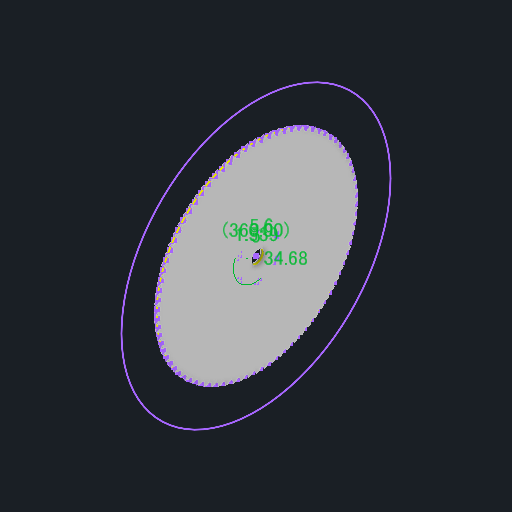
# Autodesk Inventor part: 25A80_()
Saved by Autodesk Inventor 2025.2 (Build 292293000, 293)
## iProperties
Category: PARTsolutions
Company: KANA
Created: 2025-03-15
Part Number: 25A80_()
Material: Generic
Catalog Web Link: www.cadenas.de
Description: 25A-Un-finished
Vendor: KANA
Document SubType Name: Modeling
Designer: psAdmin
Manufacturer: KANA
Mass: 58.7278 g
Surface Area: 427.105 cm^2
Volume: 58.7278 cm^3
Density: 1 g/cm^3
Appearance: PSOLRGB-175-175-175
PSOL_IDENT_0: {$CADENAS_DATA/23d-libs/kana/sprockets/chain_no_25/un_finished_sprocket_steel/a_type/25a.prj},156 {V
PSOL_IDENT_1: TYP=3D},{NB=25A80_()},{LINA=25A80},{NN=25A},{DATE=07.03.2025 00:51:20},{GEOMDATE=20.11.2024 07:31:23
PSOL_IDENT_2: },{VERSION=},{LINEID=550},{WBVAR=SURFT},{WBNUMERIC=}  {NB=25A80_()},{LINA=25A80},{KT=DUMMY},{ORDERNO=
PSOL_IDENT_3: 25A80},{TYPE=25A},{NOT=80},{NOTX=80.000},{DP=161.74},{DC=158.44},{DC2=158.44},{DO=165},{T=2.9},{DR=3
PSOL_IDENT_4: .300},{MAT=None},{MATC=},{SD=11},{SURFT=},{SURFTNB=},{DCX2=0},{CAUTION=The tooth profile in the CAD
PSOL_IDENT_5: models differ from the actual shape.}
NB: 25A80_()
NN: 25A
NT: Un-finished
NBSYN: 25A$NOT._($SURFT.)
LINA: 25A80
CATALOG: KANA
TYPE: 25A
NOT: 80
DP: 161.74
DC: 158.44
DC2: 158.44
DO: 165
T: 2.9
SD: 11
SURFT: No symbol : No
CAUTION: The tooth profile in the CAD models differ from the actual shape.
SUPPLIER: KANA
ARTICLENO: 25A80_()
BOMINFO: 25A80
CREATOR: CADENAS GmbH
Title: 25A80
Author: Cadenas PARTsolutions
Comments: Un-finished
Autodesk Inventor part; units mm, degrees
sketch "Sketch_1" plane through (0, 0, 0) normal (0, 0, 1) x (1, 0, 0)
  line L0 (2.9, 0) -> (0, 0)
  line L1 (0, 5.5) -> (2.9, 5.5)
  line L2 (2.9, 5.5) -> (2.9, 81.2642)
  arc A0 (2.9, 81.2642) -> (2.175, 82.5) centre (-0.241, 80.2521) ccw
  line L3 (2.175, 82.5) -> (0.725, 82.5)
  arc A1 (0.725, 82.5) -> (0, 81.2642) centre (3.141, 80.2521) ccw
  line L4 (0, 81.2642) -> (0, 5.5)
  constraints: 10 end point, 4 point on circle, 2 centre point
revolve "Revolution1" add sketch "Sketch_1" angle 360 about axis through (2.9, 0, 0) along (1, 0, 0)
sketch "Sketch_2" plane through (1.45, 0, 0) normal (1, 0, 0) x (0, 0, -1)
  circle A0 centre (0, -0.0001) radius 110
  arc A1 (-82.4999, 0.15) -> (-82.4999, -0.15) centre (0, -0.0001) ccw
  line L0 (-82.4999, -0.15) -> (-79.9248, -1.781)
  arc A2 (-79.8181, -4.4953) -> (-79.9248, -1.781) centre (-80.8077, -3.1749) ccw
  line L1 (-79.8181, -4.4953) -> (-82.2573, -6.3233)
  arc A3 (-82.2573, -6.3233) -> (-82.2338, -6.6224) centre (0, 0) ccw
  line L2 (-82.2338, -6.6224) -> (-79.5386, -8.0464)
  arc A4 (-79.2194, -10.7439) -> (-79.5386, -8.0464) centre (-80.3094, -9.5052) ccw
  line L3 (-79.2194, -10.7439) -> (-81.5076, -12.7577)
  arc A5 (-81.5076, -12.7577) -> (-81.4607, -13.054) centre (0, 0) ccw
  line L4 (-81.4607, -13.054) -> (-78.6621, -14.2621)
  arc A6 (-78.1322, -16.9263) -> (-78.6621, -14.2621) centre (-79.3161, -15.777) ccw
  line L5 (-78.1322, -16.9263) -> (-80.2554, -19.1134)
  arc A7 (-80.2554, -19.1134) -> (-80.1854, -19.4051) centre (0, 0) ccw
  line L6 (-80.1854, -19.4051) -> (-77.3007, -20.3899)
  arc A8 (-76.5633, -23.0043) -> (-77.3007, -20.3899) centre (-77.8338, -21.9514) ccw
  line L7 (-76.5633, -23.0043) -> (-78.5084, -25.3512)
  arc A9 (-78.5084, -25.3512) -> (-78.4157, -25.6365) centre (0, 0) ccw
  line L8 (-78.4157, -25.6365) -> (-75.4626, -26.392)
  arc A10 (-74.5224, -28.9404) -> (-75.4626, -26.392) centre (-75.8715, -27.9905) ccw
  line L9 (-74.5224, -28.9404) -> (-76.2773, -31.4327)
  arc A11 (-76.2773, -31.4327) -> (-76.1625, -31.7099) centre (0, 0) ccw
  line L10 (-76.1625, -31.7099) -> (-73.1593, -32.2313)
  arc A12 (-72.0221, -34.6982) -> (-73.1593, -32.2313) centre (-73.4415, -33.857) ccw
  line L11 (-72.0221, -34.6982) -> (-73.576, -37.3205)
  arc A13 (-73.576, -37.3205) -> (-73.4398, -37.5878) centre (0, 0) ccw
  line L12 (-73.4398, -37.5878) -> (-70.4049, -37.872)
  arc A14 (-69.0776, -40.242) -> (-70.4049, -37.872) centre (-70.5588, -39.5148) ccw
  line L13 (-69.0776, -40.242) -> (-70.4211, -42.9782)
  arc A15 (-70.4211, -42.9782) -> (-70.2643, -43.234) centre (0, 0) ccw
  line L14 (-70.2643, -43.234) -> (-67.2165, -43.2791)
  arc A16 (-65.7074, -45.5377) -> (-67.2165, -43.2791) centre (-67.2409, -44.929) ccw
  line L15 (-65.7074, -45.5377) -> (-66.832, -48.3709)
  arc A17 (-66.832, -48.3709) -> (-66.6556, -48.6136) centre (0, 0) ccw
  line L16 (-66.6556, -48.6136) -> (-63.6136, -48.4195)
  arc A18 (-61.932, -50.5527) -> (-63.6136, -48.4195) centre (-63.5086, -50.0661) ccw
  line L17 (-61.932, -50.5527) -> (-62.8308, -53.4653)
  arc A19 (-62.8308, -53.4653) -> (-62.636, -53.6934) centre (0, 0) ccw
  line L18 (-62.636, -53.6934) -> (-59.6186, -53.2613)
  arc A20 (-57.7747, -55.256) -> (-59.6186, -53.2613) centre (-59.3847, -54.8946) ccw
  line L19 (-57.7747, -55.256) -> (-58.4423, -58.2301)
  arc A21 (-58.4423, -58.2301) -> (-58.2301, -58.4423) centre (0, 0) ccw
  line L20 (-58.2301, -58.4423) -> (-55.256, -57.7747)
  arc A22 (-53.2613, -59.6186) -> (-55.256, -57.7747) centre (-54.8946, -59.3847) ccw
  line L21 (-53.2613, -59.6186) -> (-53.6934, -62.636)
  arc A23 (-53.6934, -62.636) -> (-53.4653, -62.8308) centre (0, 0) ccw
  line L22 (-53.4653, -62.8308) -> (-50.5527, -61.932)
  arc A24 (-48.4195, -63.6136) -> (-50.5527, -61.932) centre (-50.0661, -63.5086) ccw
  line L23 (-48.4195, -63.6136) -> (-48.6136, -66.6556)
  arc A25 (-48.6136, -66.6556) -> (-48.3709, -66.832) centre (0, 0) ccw
  line L24 (-48.3709, -66.832) -> (-45.5377, -65.7074)
  arc A26 (-43.2791, -67.2165) -> (-45.5377, -65.7074) centre (-44.929, -67.2409) ccw
  line L25 (-43.2791, -67.2165) -> (-43.234, -70.2643)
  arc A27 (-43.234, -70.2643) -> (-42.9782, -70.4211) centre (0, 0) ccw
  line L26 (-42.9782, -70.4211) -> (-40.242, -69.0776)
  arc A28 (-37.872, -70.4049) -> (-40.242, -69.0776) centre (-39.5148, -70.5588) ccw
  line L27 (-37.872, -70.4049) -> (-37.5878, -73.4398)
  arc A29 (-37.5878, -73.4398) -> (-37.3205, -73.576) centre (0, 0) ccw
  line L28 (-37.3205, -73.576) -> (-34.6982, -72.0221)
  arc A30 (-32.2313, -73.1593) -> (-34.6982, -72.0221) centre (-33.857, -73.4415) ccw
  line L29 (-32.2313, -73.1593) -> (-31.7099, -76.1625)
  arc A31 (-31.7099, -76.1625) -> (-31.4327, -76.2773) centre (0, 0) ccw
  line L30 (-31.4327, -76.2773) -> (-28.9404, -74.5224)
  arc A32 (-26.392, -75.4626) -> (-28.9404, -74.5224) centre (-27.9905, -75.8715) ccw
  line L31 (-26.392, -75.4626) -> (-25.6365, -78.4157)
  arc A33 (-25.6365, -78.4157) -> (-25.3512, -78.5084) centre (0, 0) ccw
  line L32 (-25.3512, -78.5084) -> (-23.0043, -76.5633)
  arc A34 (-20.3899, -77.3007) -> (-23.0043, -76.5633) centre (-21.9514, -77.8338) ccw
  line L33 (-20.3899, -77.3007) -> (-19.4051, -80.1854)
  arc A35 (-19.4051, -80.1854) -> (-19.1134, -80.2554) centre (0, 0) ccw
  line L34 (-19.1134, -80.2554) -> (-16.9263, -78.1322)
  arc A36 (-14.2621, -78.6621) -> (-16.9263, -78.1322) centre (-15.777, -79.3161) ccw
  line L35 (-14.2621, -78.6621) -> (-13.054, -81.4607)
  arc A37 (-13.054, -81.4607) -> (-12.7577, -81.5076) centre (0, 0) ccw
  line L36 (-12.7577, -81.5076) -> (-10.7439, -79.2194)
  arc A38 (-8.0464, -79.5386) -> (-10.7439, -79.2194) centre (-9.5052, -80.3094) ccw
  line L37 (-8.0464, -79.5386) -> (-6.6224, -82.2338)
  arc A39 (-6.6224, -82.2338) -> (-6.3233, -82.2573) centre (0, 0) ccw
  line L38 (-6.3233, -82.2573) -> (-4.4953, -79.8181)
  arc A40 (-1.781, -79.9248) -> (-4.4953, -79.8181) centre (-3.1749, -80.8077) ccw
  line L39 (-1.781, -79.9248) -> (-0.15, -82.4999)
  arc A41 (-0.15, -82.4999) -> (0.15, -82.4999) centre (0, 0) ccw
  line L40 (0.15, -82.4999) -> (1.781, -79.9248)
  arc A42 (4.4953, -79.8181) -> (1.781, -79.9248) centre (3.1749, -80.8077) ccw
  line L41 (4.4953, -79.8181) -> (6.3233, -82.2573)
  arc A43 (6.3233, -82.2573) -> (6.6224, -82.2338) centre (0, 0) ccw
  line L42 (6.6224, -82.2338) -> (8.0464, -79.5386)
  arc A44 (10.7439, -79.2194) -> (8.0464, -79.5386) centre (9.5052, -80.3094) ccw
  line L43 (10.7439, -79.2194) -> (12.7577, -81.5076)
  arc A45 (12.7577, -81.5076) -> (13.054, -81.4607) centre (0, 0) ccw
  line L44 (13.054, -81.4607) -> (14.2621, -78.6621)
  arc A46 (16.9263, -78.1322) -> (14.2621, -78.6621) centre (15.777, -79.3161) ccw
  line L45 (16.9263, -78.1322) -> (19.1134, -80.2554)
  arc A47 (19.1134, -80.2554) -> (19.4051, -80.1854) centre (0, 0) ccw
  line L46 (19.4051, -80.1854) -> (20.3899, -77.3007)
  arc A48 (23.0043, -76.5633) -> (20.3899, -77.3007) centre (21.9514, -77.8338) ccw
  line L47 (23.0043, -76.5633) -> (25.3512, -78.5084)
  arc A49 (25.3512, -78.5084) -> (25.6365, -78.4157) centre (0, 0) ccw
  line L48 (25.6365, -78.4157) -> (26.392, -75.4626)
  arc A50 (28.9404, -74.5224) -> (26.392, -75.4626) centre (27.9905, -75.8715) ccw
  line L49 (28.9404, -74.5224) -> (31.4327, -76.2773)
  arc A51 (31.4327, -76.2773) -> (31.7099, -76.1625) centre (0, 0) ccw
  line L50 (31.7099, -76.1625) -> (32.2313, -73.1593)
  arc A52 (34.6982, -72.0221) -> (32.2313, -73.1593) centre (33.857, -73.4415) ccw
  line L51 (34.6982, -72.0221) -> (37.3205, -73.576)
  arc A53 (37.3205, -73.576) -> (37.5878, -73.4398) centre (0, 0) ccw
  line L52 (37.5878, -73.4398) -> (37.872, -70.4049)
  arc A54 (40.242, -69.0776) -> (37.872, -70.4049) centre (39.5148, -70.5588) ccw
  line L53 (40.242, -69.0776) -> (42.9782, -70.4211)
  arc A55 (42.9782, -70.4211) -> (43.234, -70.2643) centre (0, 0) ccw
  line L54 (43.234, -70.2643) -> (43.2791, -67.2165)
  arc A56 (45.5377, -65.7074) -> (43.2791, -67.2165) centre (44.929, -67.2409) ccw
  line L55 (45.5377, -65.7074) -> (48.3709, -66.832)
  arc A57 (48.3709, -66.832) -> (48.6136, -66.6556) centre (0, 0) ccw
  line L56 (48.6136, -66.6556) -> (48.4195, -63.6136)
  arc A58 (50.5527, -61.932) -> (48.4195, -63.6136) centre (50.0661, -63.5086) ccw
  line L57 (50.5527, -61.932) -> (53.4653, -62.8308)
  arc A59 (53.4653, -62.8308) -> (53.6934, -62.636) centre (0, 0) ccw
  line L58 (53.6934, -62.636) -> (53.2613, -59.6186)
  arc A60 (55.256, -57.7747) -> (53.2613, -59.6186) centre (54.8946, -59.3847) ccw
  line L59 (55.256, -57.7747) -> (58.2301, -58.4423)
  arc A61 (58.2301, -58.4423) -> (58.4423, -58.2301) centre (0, 0) ccw
  line L60 (58.4423, -58.2301) -> (57.7747, -55.256)
  arc A62 (59.6186, -53.2613) -> (57.7747, -55.256) centre (59.3847, -54.8946) ccw
  line L61 (59.6186, -53.2613) -> (62.636, -53.6934)
  arc A63 (62.636, -53.6934) -> (62.8308, -53.4653) centre (0, 0) ccw
  line L62 (62.8308, -53.4653) -> (61.9319, -50.5527)
  arc A64 (63.6136, -48.4195) -> (61.9319, -50.5527) centre (63.5086, -50.0661) ccw
  line L63 (63.6136, -48.4195) -> (66.6556, -48.6136)
  arc A65 (66.6556, -48.6136) -> (66.832, -48.3709) centre (0, 0) ccw
  line L64 (66.832, -48.3709) -> (65.7074, -45.5377)
  arc A66 (67.2165, -43.2791) -> (65.7074, -45.5377) centre (67.2409, -44.929) ccw
  line L65 (67.2165, -43.2791) -> (70.2643, -43.234)
  arc A67 (70.2643, -43.234) -> (70.4211, -42.9782) centre (0, 0) ccw
  line L66 (70.4211, -42.9782) -> (69.0776, -40.242)
  arc A68 (70.4049, -37.872) -> (69.0776, -40.242) centre (70.5588, -39.5148) ccw
  line L67 (70.4049, -37.872) -> (73.4398, -37.5878)
  arc A69 (73.4398, -37.5878) -> (73.576, -37.3205) centre (0, 0) ccw
  line L68 (73.576, -37.3205) -> (72.0221, -34.6982)
  arc A70 (73.1593, -32.2313) -> (72.0221, -34.6982) centre (73.4415, -33.857) ccw
  line L69 (73.1593, -32.2313) -> (76.1625, -31.7099)
  arc A71 (76.1625, -31.7099) -> (76.2773, -31.4327) centre (0, 0) ccw
  line L70 (76.2773, -31.4327) -> (74.5224, -28.9404)
  arc A72 (75.4626, -26.392) -> (74.5224, -28.9404) centre (75.8715, -27.9905) ccw
  line L71 (75.4626, -26.392) -> (78.4157, -25.6365)
  arc A73 (78.4157, -25.6365) -> (78.5084, -25.3512) centre (0, 0) ccw
  line L72 (78.5084, -25.3512) -> (76.5633, -23.0043)
  arc A74 (77.3007, -20.3899) -> (76.5633, -23.0043) centre (77.8338, -21.9514) ccw
  line L73 (77.3007, -20.3899) -> (80.1854, -19.4051)
  arc A75 (80.1854, -19.4051) -> (80.2554, -19.1134) centre (0, 0) ccw
  line L74 (80.2554, -19.1134) -> (78.1322, -16.9263)
  arc A76 (78.6621, -14.2621) -> (78.1322, -16.9263) centre (79.3161, -15.777) ccw
  line L75 (78.6621, -14.2621) -> (81.4607, -13.054)
  arc A77 (81.4607, -13.054) -> (81.5076, -12.7577) centre (0, 0) ccw
  line L76 (81.5076, -12.7577) -> (79.2194, -10.7439)
  arc A78 (79.5386, -8.0464) -> (79.2194, -10.7439) centre (80.3094, -9.5052) ccw
  line L77 (79.5386, -8.0464) -> (82.2338, -6.6224)
  arc A79 (82.2338, -6.6224) -> (82.2573, -6.3233) centre (0, 0) ccw
  line L78 (82.2573, -6.3233) -> (79.8181, -4.4953)
  arc A80 (79.9248, -1.781) -> (79.8181, -4.4953) centre (80.8077, -3.1749) ccw
  line L79 (79.9248, -1.781) -> (82.4999, -0.15)
  arc A81 (82.4999, -0.15) -> (82.4999, 0.15) centre (0, 0) ccw
  line L80 (82.4999, 0.15) -> (79.9248, 1.781)
  arc A82 (79.8181, 4.4953) -> (79.9248, 1.781) centre (80.8077, 3.1749) ccw
  line L81 (79.8181, 4.4953) -> (82.2573, 6.3233)
  arc A83 (82.2573, 6.3233) -> (82.2338, 6.6224) centre (0, 0) ccw
  line L82 (82.2338, 6.6224) -> (79.5386, 8.0464)
  arc A84 (79.2194, 10.7439) -> (79.5386, 8.0464) centre (80.3094, 9.5052) ccw
  line L83 (79.2194, 10.7439) -> (81.5076, 12.7577)
  arc A85 (81.5076, 12.7577) -> (81.4607, 13.054) centre (0, 0) ccw
  line L84 (81.4607, 13.054) -> (78.6621, 14.2621)
  arc A86 (78.1322, 16.9263) -> (78.6621, 14.2621) centre (79.3161, 15.777) ccw
  line L85 (78.1322, 16.9263) -> (80.2554, 19.1134)
  arc A87 (80.2554, 19.1134) -> (80.1854, 19.4051) centre (0, 0) ccw
  line L86 (80.1854, 19.4051) -> (77.3007, 20.3899)
  arc A88 (76.5633, 23.0043) -> (77.3007, 20.3899) centre (77.8338, 21.9514) ccw
  line L87 (76.5633, 23.0043) -> (78.5084, 25.3512)
  arc A89 (78.5084, 25.3512) -> (78.4157, 25.6365) centre (0, 0) ccw
  line L88 (78.4157, 25.6365) -> (75.4626, 26.392)
  arc A90 (74.5224, 28.9404) -> (75.4626, 26.392) centre (75.8715, 27.9905) ccw
  line L89 (74.5224, 28.9404) -> (76.2773, 31.4327)
  arc A91 (76.2773, 31.4327) -> (76.1625, 31.7099) centre (0, 0) ccw
  line L90 (76.1625, 31.7099) -> (73.1593, 32.2313)
  arc A92 (72.0221, 34.6982) -> (73.1593, 32.2313) centre (73.4415, 33.857) ccw
  line L91 (72.0221, 34.6982) -> (73.576, 37.3205)
  arc A93 (73.576, 37.3205) -> (73.4398, 37.5878) centre (0, 0) ccw
  line L92 (73.4398, 37.5878) -> (70.4049, 37.872)
  arc A94 (69.0776, 40.242) -> (70.4049, 37.872) centre (70.5588, 39.5148) ccw
  line L93 (69.0776, 40.242) -> (70.4211, 42.9782)
  arc A95 (70.4211, 42.9782) -> (70.2643, 43.234) centre (0, 0) ccw
  line L94 (70.2643, 43.234) -> (67.2165, 43.2791)
  arc A96 (65.7074, 45.5377) -> (67.2165, 43.2791) centre (67.2409, 44.929) ccw
  line L95 (65.7074, 45.5377) -> (66.832, 48.3709)
  arc A97 (66.832, 48.3709) -> (66.6556, 48.6136) centre (0, 0) ccw
  line L96 (66.6556, 48.6136) -> (63.6136, 48.4195)
  arc A98 (61.932, 50.5527) -> (63.6136, 48.4195) centre (63.5086, 50.0661) ccw
  line L97 (61.932, 50.5527) -> (62.8308, 53.4653)
  arc A99 (62.8308, 53.4653) -> (62.636, 53.6934) centre (0, 0) ccw
  line L98 (62.636, 53.6934) -> (59.6186, 53.2613)
  arc A100 (57.7747, 55.256) -> (59.6186, 53.2613) centre (59.3847, 54.8946) ccw
  line L99 (57.7747, 55.256) -> (58.4423, 58.2301)
  arc A101 (58.4423, 58.2301) -> (58.2301, 58.4423) centre (0, 0) ccw
  line L100 (58.2301, 58.4423) -> (55.256, 57.7747)
  arc A102 (53.2613, 59.6186) -> (55.256, 57.7747) centre (54.8946, 59.3847) ccw
  line L101 (53.2613, 59.6186) -> (53.6934, 62.636)
  arc A103 (53.6934, 62.636) -> (53.4653, 62.8308) centre (0, 0) ccw
  line L102 (53.4653, 62.8308) -> (50.5527, 61.932)
  arc A104 (48.4195, 63.6136) -> (50.5527, 61.932) centre (50.0661, 63.5086) ccw
  line L103 (48.4195, 63.6136) -> (48.6136, 66.6556)
  arc A105 (48.6136, 66.6556) -> (48.3709, 66.832) centre (0, 0) ccw
  line L104 (48.3709, 66.832) -> (45.5377, 65.7074)
  arc A106 (43.2791, 67.2165) -> (45.5377, 65.7074) centre (44.929, 67.2409) ccw
  line L105 (43.2791, 67.2165) -> (43.234, 70.2643)
  arc A107 (43.234, 70.2643) -> (42.9782, 70.4211) centre (0, 0) ccw
  line L106 (42.9782, 70.4211) -> (40.242, 69.0776)
  arc A108 (37.872, 70.4049) -> (40.242, 69.0776) centre (39.5148, 70.5588) ccw
  line L107 (37.872, 70.4049) -> (37.5878, 73.4398)
  arc A109 (37.5878, 73.4398) -> (37.3205, 73.576) centre (0, 0) ccw
  line L108 (37.3205, 73.576) -> (34.6982, 72.0221)
  arc A110 (32.2313, 73.1593) -> (34.6982, 72.0221) centre (33.857, 73.4415) ccw
  line L109 (32.2313, 73.1593) -> (31.7099, 76.1625)
  arc A111 (31.7099, 76.1625) -> (31.4327, 76.2773) centre (0, 0) ccw
  line L110 (31.4327, 76.2773) -> (28.9404, 74.5224)
  arc A112 (26.392, 75.4626) -> (28.9404, 74.5224) centre (27.9905, 75.8715) ccw
  line L111 (26.392, 75.4626) -> (25.6365, 78.4157)
  arc A113 (25.6365, 78.4157) -> (25.3512, 78.5084) centre (0, 0) ccw
  line L112 (25.3512, 78.5084) -> (23.0043, 76.5633)
  arc A114 (20.3899, 77.3007) -> (23.0043, 76.5633) centre (21.9514, 77.8338) ccw
  line L113 (20.3899, 77.3007) -> (19.4051, 80.1854)
  arc A115 (19.4051, 80.1854) -> (19.1134, 80.2554) centre (0, 0) ccw
  line L114 (19.1134, 80.2554) -> (16.9263, 78.1322)
  arc A116 (14.2621, 78.6621) -> (16.9263, 78.1322) centre (15.777, 79.3161) ccw
  line L115 (14.2621, 78.6621) -> (13.054, 81.4607)
  arc A117 (13.054, 81.4607) -> (12.7577, 81.5076) centre (0, 0) ccw
  line L116 (12.7577, 81.5076) -> (10.7439, 79.2194)
  arc A118 (8.0464, 79.5386) -> (10.7439, 79.2194) centre (9.5052, 80.3094) ccw
  line L117 (8.0464, 79.5386) -> (6.6224, 82.2338)
  arc A119 (6.6224, 82.2338) -> (6.3233, 82.2573) centre (0, 0) ccw
  line L118 (6.3233, 82.2573) -> (4.4953, 79.8181)
  arc A120 (1.781, 79.9248) -> (4.4953, 79.8181) centre (3.1749, 80.8077) ccw
  line L119 (1.781, 79.9248) -> (0.15, 82.4999)
  arc A121 (0.15, 82.4999) -> (-0.15, 82.4999) centre (0, 0) ccw
  line L120 (-0.15, 82.4999) -> (-1.781, 79.9248)
  arc A122 (-4.4953, 79.8181) -> (-1.781, 79.9248) centre (-3.1749, 80.8077) ccw
  line L121 (-4.4953, 79.8181) -> (-6.3233, 82.2573)
  arc A123 (-6.3233, 82.2573) -> (-6.6224, 82.2338) centre (0, 0) ccw
  line L122 (-6.6224, 82.2338) -> (-8.0464, 79.5386)
  arc A124 (-10.7439, 79.2194) -> (-8.0464, 79.5386) centre (-9.5052, 80.3094) ccw
  line L123 (-10.7439, 79.2194) -> (-12.7577, 81.5076)
  arc A125 (-12.7577, 81.5076) -> (-13.054, 81.4607) centre (0, 0) ccw
  line L124 (-13.054, 81.4607) -> (-14.2621, 78.6621)
  arc A126 (-16.9263, 78.1322) -> (-14.2621, 78.6621) centre (-15.777, 79.3161) ccw
  line L125 (-16.9263, 78.1322) -> (-19.1134, 80.2554)
  arc A127 (-19.1134, 80.2554) -> (-19.4051, 80.1854) centre (0, 0) ccw
  line L126 (-19.4051, 80.1854) -> (-20.3899, 77.3007)
  arc A128 (-23.0043, 76.5633) -> (-20.3899, 77.3007) centre (-21.9514, 77.8338) ccw
  line L127 (-23.0043, 76.5633) -> (-25.3512, 78.5084)
  arc A129 (-25.3512, 78.5084) -> (-25.6365, 78.4157) centre (0, 0) ccw
  line L128 (-25.6365, 78.4157) -> (-26.392, 75.4626)
  arc A130 (-28.9404, 74.5224) -> (-26.392, 75.4626) centre (-27.9905, 75.8715) ccw
  line L129 (-28.9404, 74.5224) -> (-31.4327, 76.2773)
  arc A131 (-31.4327, 76.2773) -> (-31.7099, 76.1625) centre (0, 0) ccw
  line L130 (-31.7099, 76.1625) -> (-32.2313, 73.1593)
  arc A132 (-34.6982, 72.0221) -> (-32.2313, 73.1593) centre (-33.857, 73.4415) ccw
  line L131 (-34.6982, 72.0221) -> (-37.3205, 73.576)
  arc A133 (-37.3205, 73.576) -> (-37.5878, 73.4398) centre (0, 0) ccw
  line L132 (-37.5878, 73.4398) -> (-37.872, 70.4049)
  arc A134 (-40.242, 69.0776) -> (-37.872, 70.4049) centre (-39.5148, 70.5588) ccw
  line L133 (-40.242, 69.0776) -> (-42.9782, 70.4211)
  arc A135 (-42.9782, 70.4211) -> (-43.234, 70.2643) centre (0, 0) ccw
  line L134 (-43.234, 70.2643) -> (-43.2791, 67.2165)
  arc A136 (-45.5377, 65.7074) -> (-43.2791, 67.2165) centre (-44.929, 67.2409) ccw
  line L135 (-45.5377, 65.7074) -> (-48.3709, 66.832)
  arc A137 (-48.3709, 66.832) -> (-48.6136, 66.6556) centre (0, 0) ccw
  line L136 (-48.6136, 66.6556) -> (-48.4195, 63.6136)
  arc A138 (-50.5527, 61.932) -> (-48.4195, 63.6136) centre (-50.0661, 63.5086) ccw
  line L137 (-50.5527, 61.932) -> (-53.4653, 62.8308)
  arc A139 (-53.4653, 62.8308) -> (-53.6934, 62.636) centre (0, 0) ccw
  line L138 (-53.6934, 62.636) -> (-53.2613, 59.6186)
  arc A140 (-55.256, 57.7747) -> (-53.2613, 59.6186) centre (-54.8946, 59.3847) ccw
  line L139 (-55.256, 57.7747) -> (-58.2301, 58.4423)
  arc A141 (-58.2301, 58.4423) -> (-58.4423, 58.2301) centre (0, 0) ccw
  line L140 (-58.4423, 58.2301) -> (-57.7747, 55.256)
  arc A142 (-59.6186, 53.2613) -> (-57.7747, 55.256) centre (-59.3847, 54.8946) ccw
  line L141 (-59.6186, 53.2613) -> (-62.636, 53.6934)
  arc A143 (-62.636, 53.6934) -> (-62.8308, 53.4653) centre (0, 0) ccw
  line L142 (-62.8308, 53.4653) -> (-61.932, 50.5527)
  arc A144 (-63.6136, 48.4195) -> (-61.932, 50.5527) centre (-63.5086, 50.0661) ccw
  line L143 (-63.6136, 48.4195) -> (-66.6556, 48.6136)
  arc A145 (-66.6556, 48.6136) -> (-66.832, 48.3709) centre (0, 0) ccw
  line L144 (-66.832, 48.3709) -> (-65.7074, 45.5377)
  arc A146 (-67.2165, 43.2791) -> (-65.7074, 45.5377) centre (-67.2409, 44.929) ccw
  line L145 (-67.2165, 43.2791) -> (-70.2643, 43.234)
  arc A147 (-70.2643, 43.234) -> (-70.4211, 42.9782) centre (0, 0) ccw
  line L146 (-70.4211, 42.9782) -> (-69.0776, 40.242)
  arc A148 (-70.4049, 37.872) -> (-69.0776, 40.242) centre (-70.5588, 39.5148) ccw
  line L147 (-70.4049, 37.872) -> (-73.4398, 37.5878)
  arc A149 (-73.4398, 37.5878) -> (-73.576, 37.3205) centre (0, 0) ccw
  line L148 (-73.576, 37.3205) -> (-72.0221, 34.6982)
  arc A150 (-73.1593, 32.2313) -> (-72.0221, 34.6982) centre (-73.4415, 33.857) ccw
  line L149 (-73.1593, 32.2313) -> (-76.1625, 31.7099)
  arc A151 (-76.1625, 31.7099) -> (-76.2773, 31.4327) centre (0, 0) ccw
  line L150 (-76.2773, 31.4327) -> (-74.5224, 28.9404)
  arc A152 (-75.4626, 26.392) -> (-74.5224, 28.9404) centre (-75.8715, 27.9905) ccw
  line L151 (-75.4626, 26.392) -> (-78.4157, 25.6365)
  arc A153 (-78.4157, 25.6365) -> (-78.5084, 25.3512) centre (0, 0) ccw
  line L152 (-78.5084, 25.3512) -> (-76.5633, 23.0043)
  arc A154 (-77.3007, 20.3899) -> (-76.5633, 23.0043) centre (-77.8338, 21.9514) ccw
  line L153 (-77.3007, 20.3899) -> (-80.1854, 19.4051)
  arc A155 (-80.1854, 19.4051) -> (-80.2554, 19.1134) centre (0, 0) ccw
  line L154 (-80.2554, 19.1134) -> (-78.1322, 16.9263)
  arc A156 (-78.6621, 14.2621) -> (-78.1322, 16.9263) centre (-79.3161, 15.777) ccw
  line L155 (-78.6621, 14.2621) -> (-81.4607, 13.054)
  arc A157 (-81.4607, 13.054) -> (-81.5076, 12.7577) centre (0, 0) ccw
  line L156 (-81.5076, 12.7577) -> (-79.2194, 10.7439)
  arc A158 (-79.5386, 8.0464) -> (-79.2194, 10.7439) centre (-80.3094, 9.5052) ccw
  line L157 (-79.5386, 8.0464) -> (-82.2338, 6.6224)
  arc A159 (-82.2338, 6.6224) -> (-82.2573, 6.3233) centre (0, 0) ccw
  line L158 (-82.2573, 6.3233) -> (-79.8181, 4.4953)
  arc A160 (-79.9248, 1.781) -> (-79.8181, 4.4953) centre (-80.8077, 3.1749) ccw
  line L159 (-79.9248, 1.781) -> (-82.4999, 0.15)
  circle A161 centre (0, 0) radius 17.34
  circle A162 centre (0, 0) radius 81.2642 projected
  circle A163 centre (0, 0) radius 5.5 projected
  circle A164 centre (0, 0) radius 18.4198
  circle A165 centre (0, 18.4198) radius 2.8
  line L160 (-2.5, 17.1588) -> (2.5, 17.1588)
  line L161 (0, 15.6198) -> (0, 17.1588)
  circle A166 centre (-15.952, 9.2099) radius 2.8
  circle A167 centre (-15.952, -9.2099) radius 2.8
  circle A168 centre (0, -18.4198) radius 2.8
  circle A169 centre (15.952, -9.2099) radius 2.8
  circle A170 centre (15.952, 9.2099) radius 2.8
  point P0 (-16.11, 6.4144)
  point P1 (-13.61, 10.7445)
  point P2 (-13.5271, 7.8099)
  point P3 (-13.61, -10.7445)
  point P4 (-16.11, -6.4144)
  point P5 (-13.5271, -7.8099)
  point P6 (2.5, -17.1588)
  point P7 (-2.5, -17.1588)
  point P8 (0, -15.6198)
  point P9 (16.11, -6.4144)
  point P10 (13.61, -10.7445)
  point P11 (13.5271, -7.8099)
  point P12 (13.61, 10.7445)
  point P13 (16.11, 6.4144)
  point P14 (13.5271, 7.8099)
  dimension "d5" = 34.68
  dimension "d9" = 5.6
  dimension "d10" = 5
  dimension "d11" = 1.5391
  dimension "d14" = 360
  constraints: 340 point on circle, 324 end point, 168 centre point, 5 coincident, 1 concentric, 1 midpoint, 34 other
  measures "d5" diameter of A161
  measures "d9" diameter of A165
  measures "d10" distance of L160.start L160.end
  measures "d11" distance of L161.start L161.end
extrude "Extrusion1" cut sketch "Sketch_2" along normal mid plane 3.3 contours A0 | A162 L158 A160 L159 | L0 A2 L1 A162 | A162 L156 A158 L157 | L2 A4 L3 A162 | A162 L154 A156 L155 | L4 A6 L5 A162 | A162 L152 A154 L153 | L6 A8 L7 A162 | A162 L150 A152 L151 | L8 A10 L9 A162 | A162 L148 A150 L149 | L10 A12 L11 A162 | A162 L146 A148 L147 | L12 A14 L13 A162 | A162 L144 A146 L145 | L14 A16 L15 A162 | A162 L142 A144 L143 | L16 A18 L17 A162 | A162 L140 A142 L141 | L18 A20 L19 A162 | A162 L138 A140 L139 | L20 A22 L21 A162 | A162 L136 A138 L137 | L22 A24 L23 A162 | A162 L134 A136 L135 | L24 A26 L25 A162 | A162 L132 A134 L133 | L26 A28 L27 A162 | A162 L130 A132 L131 | L28 A30 L29 A162 | A162 L128 A130 L129 | L30 A32 L31 A162 | A162 L126 A128 L127 | L32 A34 L33 A162 | A162 L124 A126 L125 | L34 A36 L35 A162 | A162 L122 A124 L123 | L36 A38 L37 A162 | A162 L120 A122 L121 | L38 A40 L39 A162 | A162 L118 A120 L119 | L40 A42 L41 A162 | A162 L116 A118 L117 | L42 A44 L43 A162 | A162 L114 A116 L115 | L44 A46 L45 A162 | A162 L112 A114 L113 | L46 A48 L47 A162 | A162 L110 A112 L111 | L48 A50 L49 A162 | A162 L108 A110 L109 | L50 A52 L51 A162 | A162 L106 A108 L107 | L52 A54 L53 A162 | A162 L104 A106 L105 | L54 A56 L55 A162 | A162 L102 A104 L103 | L56 A58 L57 A162 | A162 L100 A102 L101 | L58 A60 L59 A162 | A162 L98 A100 L99 | L60 A62 L61 A162 | A162 L96 A98 L97 | L62 A64 L63 A162 | A162 L94 A96 L95 | L64 A66 L65 A162 | A162 L92 A94 L93 | L66 A68 L67 A162 | A162 L90 A92 L91 | L68 A70 L69 A162 | A162 L88 A90 L89 | L70 A72 L71 A162 | A162 L86 A88 L87 | L72 A74 L73 A162 | A162 L84 A86 L85 | L74 A76 L75 A162 | A162 L82 A84 L83 | L76 A78 L77 A162 | A162 L80 A82 L81 | L78 A80 L79 A162
ref_plane "Body_XY" through (0, 0, 0) normal (1, 0, 0) x (0, 0, -1)
ref_plane "Body_YZ" through (0, 0, 0) normal (0, 0, -1) x (0, 1, 0)
ref_plane "Body_ZX" through (0, 0, 0) normal (0, 1, 0) x (1, 0, 0)
body "Solid1"
